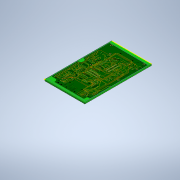
# Autodesk Inventor part: PCB
Saved by Autodesk Inventor 2021 (Build 250183000, 183)
## iProperties
Created: 2023-04-06
Part Number: PCB
Material: Generic
Document SubType Name: Modeling
Designer: EF0481
Density: 1 g/cm^3
Appearance: Default
Author: EF0481
Autodesk Inventor part; units mm, degrees
ref_plane "YZ Plane" through (0, 0, 0) normal (1, 0, 0) x (0, 1, 0)
ref_plane "XZ Plane" through (0, 0, 0) normal (0, 1, 0) x (-1, 0, 0)
ref_plane "XY Plane" through (0, 0, 0) normal (0, 0, 1) x (1, 0, 0)
sketch "Sketch1" plane through (0, 0, 0) normal (0, 0, 1) x (1, 0, 0)
  line L0 (0, 0) -> (45, 0)
  line L1 (45, 0) -> (45, 1.55)
  line L2 (45, 1.55) -> (0, 1.55)
  line L3 (0, 1.55) -> (0, 0)
  dimension "d0" = 45
  dimension "d1" = 1.55
  constraints: 8 end point, 2 parallel, 1 horizontal, 1 perpendicular
  measures "d0" distance of L2.end L1.end
  measures "d1" distance of L1.end L0.end
extrude "Extrusion1" add sketch "Sketch1" against normal blind 75
sketch "Sketch2" plane through (0, 1.55, 0) normal (0, 1, 0) x (1, 0, 0)
  line L0 (45, 75) -> (0, 75) projected
  line L1 (0.7554, 1.8482) -> (0.7554, 71.8482) construction
  line L2 (0.7554, 71.8482) -> (44.1554, 71.8482) construction
  line L3 (44.1554, 71.8482) -> (44.1554, 1.8482) construction
  line L4 (44.1554, 1.8482) -> (0.7554, 1.8482) construction
  point P0 (0, 0)
  constraints: 2 other
body "Solid1"
